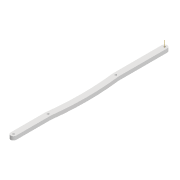
# Autodesk Inventor part: Part_3
Saved by Autodesk Inventor 2022 (Build 260153000, 153)
## iProperties
Created: 2022-04-22
Part Number: Part_3
Material: Generic
Document SubType Name: Modeling
Designer: dell
Density: 1 g/cm^3
Appearance: Default
Mass: 3.16709 g
Surface Area: 28.078 cm^2
Volume: 3.16709 cm^3
Author: dell
Autodesk Inventor part; units mm, degrees
ref_plane "YZ Plane" through (0, 0, 0) normal (1, 0, 0) x (0, 1, 0)
ref_plane "XZ Plane" through (0, 0, 0) normal (0, 1, 0) x (-1, 0, 0)
ref_plane "XY Plane" through (0, 0, 0) normal (0, 0, 1) x (1, 0, 0)
sketch "Sketch1" plane through (0, 0, 0) normal (0, 1, 0) x (-1, 0, 0)
  line L0 (0, 0) -> (0, -163.527) construction
  line L1 (3, 0) -> (3, -163.527)
  line L2 (-3, -163.527) -> (-3, 0)
  arc A0 (3, 0) -> (-3, 0) centre (0, 0) ccw
  arc A1 (-3, -163.527) -> (3, -163.527) centre (0, -163.527) ccw
  circle A2 centre (0, 0) radius 1.1
  circle A3 centre (0, -163.527) radius 1.1
  circle A4 centre (0, -37.565) radius 1.1
  circle A5 centre (0, -110.762) radius 1.1
  arc A6 (3, -37.565) -> (3, -110.762) centre (300.7592, -74.1635) ccw
  arc A7 (-3, -37.565) -> (-3, -110.762) centre (294.7592, -74.1635) ccw
  point P0 (0, -81.7635)
  dimension "d0" = 2.2
  dimension "d1" = 2.2
  dimension "d2" = 6
  dimension "d3" = 163.527
  dimension "d4" = 2.2
  dimension "d5" = 37.565
  dimension "d8" = 2.2
  dimension "d9" = 110.762
  dimension "d10" = 300
  dimension "d11" = 300
  constraints: 8 centre point, 8 end point, 8 point on circle, 6 point on line, 4 horizontal alignment, 4 tangent, 2 coincident, 1 midpoint, 1 parallel, 1 vertical
  measures "d0" diameter of A2
  measures "d1" diameter of A3
  measures "d2" distance between parallel lines of L2 L1
  measures "d3" distance of L0.end L0.start
  measures "d4" diameter of A4
  measures "d5" distance of L0.start A4.centre
  measures "d8" diameter of A5
  measures "d9" distance of L0.start A5.centre
  measures "d10" radius of A6
  measures "d11" radius of A7
extrude "Extrusion1" add sketch "Sketch1" along normal blind 4 contours L1 A6 A1 L2 A0 | L2 A7
body "Solid1"
